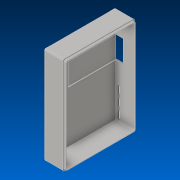
# Autodesk Inventor part: Bottom
Saved by Autodesk Inventor 2016 (Build 200138000, 138)
## iProperties
Created: 2015-08-21
Part Number: Bottom
Material: Generic
Document SubType Name: Modeling
Designer: Moffitt
Density: 1 g/cm^3
Appearance: Default
Author: Moffitt
Autodesk Inventor part; units mm, degrees
ref_plane "YZ Plane" through (0, 0, 0) normal (1, 0, 0) x (0, 1, 0)
ref_plane "XZ Plane" through (0, 0, 0) normal (0, 1, 0) x (-1, 0, 0)
ref_plane "XY Plane" through (0, 0, 0) normal (0, 0, 1) x (1, 0, 0)
sketch "Very Bottom" plane through (0, 0, 0) normal (1, 0, 0) x (0, 1, 0)
  line L0 (98.706, 61.2459) -> (-91.294, 61.2459)
  line L1 (-91.294, 61.2459) -> (-91.294, -78.7541)
  line L2 (-91.294, -78.7541) -> (98.706, -78.7541)
  line L3 (98.706, -78.7541) -> (98.706, 61.2459)
  point P0 (0, 0)
  dimension "d4" = 140
  dimension "d5" = 190
  constraints: 8 end point, 2 parallel, 1 horizontal, 1 perpendicular
  measures "d4" distance of L2.end L0.start
  measures "d5" distance of L1.end L2.end
extrude "Extrusion1" add sketch "Very Bottom" along normal blind 4
sketch "Walls A" plane through (4, 0, 0) normal (1, 0, 0) x (0, 0, -1)
  line L0 (-58.2459, 95.706) -> (75.7541, 95.706)
  line L1 (75.7541, 95.706) -> (75.7541, -88.294)
  line L2 (75.7541, -88.294) -> (-58.2459, -88.294)
  line L3 (-58.2459, -88.294) -> (-58.2459, 95.706)
  line L4 (78.7541, 98.706) -> (-61.2459, 98.706) projected
  line L5 (-61.2459, -91.294) -> (78.7541, -91.294) projected
  line L6 (-61.2459, 98.706) -> (-61.2459, -91.294) projected
  line L7 (78.7541, -91.294) -> (78.7541, 98.706) projected
  point P0 (0, 0)
  dimension "d6" = 3
  dimension "d7" = 3
  dimension "d8" = 3
  dimension "d9" = 3
  constraints: 8 end point, 2 parallel, 1 horizontal, 1 perpendicular
  measures "d6" distance between parallel lines of L4 L0
  measures "d7" distance between parallel lines of L5 L2
  measures "d8" distance between parallel lines of L3 L6
  measures "d9" distance between parallel lines of L7 L1
extrude "Walls" add sketch "Walls A" along normal blind 38
sketch "Back Panel" plane through (0, -91.294, -78.7541) normal (0, 0, -1) x (-1, 0, 0)
  line L0 (0, 0) -> (-42, 0) projected
  line L1 (-4, 3) -> (-4, 187) projected
  line L2 (-4, 103.5669) -> (-19, 103.5669)
  line L3 (-19, 103.5669) -> (-19, 147.5669)
  line L4 (-19, 147.5669) -> (-4, 147.5669)
  line L5 (-4, 147.5669) -> (-4, 103.5669)
  line L6 (-4, 147.5669) -> (0, 147.5669)
  line L7 (0, 147.5669) -> (0, 103.5669)
  line L8 (0, 103.5669) -> (-4, 103.5669)
  line L9 (-4, 103.5669) -> (-4, 147.5669)
  point P0 (0, 91.294)
  dimension "d33" = 44
  dimension "d34" = 15
  dimension "d52" = 4
  constraints: 16 end point, 4 parallel, 2 horizontal, 2 perpendicular, 1 point on line
  measures "d33" distance of L2.end L3.end
  measures "d34" distance of L3.end L4.end
  measures "d52" distance of L4.end L6.end
fillet "Fillet1" radius 3 12 edges at (21, 98.706, -78.7541) (0, 3.706, -78.7541) (21, -91.294, -78.7541) (0, -91.294, -8.7541) (21, -91.294, 61.2459) (0, 3.706, 61.2459) (21, 98.706, 61.2459) (23, 95.706, 58.2459) (23, 95.706, -75.7541) (23, -88.294, -75.7541) (23, -88.294, 58.2459) (0, 98.706, -8.7541)
sketch "Sketch9" plane through (3, 98.706, -75.7541) normal (0, 1, 0) x (1, 0, 0)
  line L0 (-3, 0) -> (-3, -134) projected
  line L1 (-3, -132.5) -> (-1.5, -132.5)
  line L2 (-1.5, -132.5) -> (-1.5, -130.5)
  line L3 (-1.5, -130.5) -> (-3, -130.5)
  line L4 (-3, -130.5) -> (-3, -132.5)
  line L5 (-3, -128.5) -> (-1.5, -128.5)
  line L6 (-1.5, -128.5) -> (-1.5, -126.5)
  line L7 (-1.5, -126.5) -> (-3, -126.5)
  line L8 (-3, -126.5) -> (-3, -128.5)
  line L9 (-3, -1.5) -> (-1.5, -1.5)
  line L10 (-1.5, -1.5) -> (-1.5, -3.5)
  line L11 (-1.5, -3.5) -> (-3, -3.5)
  line L12 (-3, -3.5) -> (-3, -1.5)
  line L13 (-3, -5.5) -> (-1.5, -5.5)
  line L14 (-1.5, -5.5) -> (-1.5, -7.5)
  line L15 (-1.5, -7.5) -> (-3, -7.5)
  line L16 (-3, -7.5) -> (-3, -5.5)
  point P0 (-3, -75.7541)
  dimension "d66" = 1.5
  dimension "d67" = 1.5
  dimension "d68" = 2
  dimension "d69" = 2
  dimension "d70" = 2
  dimension "d71" = 2
  dimension "d72" = 2
  dimension "d73" = 1.5
  dimension "d74" = 2
  dimension "d75" = 1.5
  dimension "d76" = 1.5
  constraints: 32 end point, 8 parallel, 5 point on line, 4 horizontal, 4 perpendicular
  measures "d66" distance of L14.end L15.end
  measures "d67" distance of L10.end L11.end
  measures "d68" distance of L9.end L10.end
  measures "d69" distance of L13.end L14.end
  measures "d70" distance between parallel lines of L11 L13
  measures "d71" distance of L1.end L2.end
  measures "d72" distance of L5.end L6.end
  measures "d73" distance from line of L0.end L1
  measures "d74" distance between parallel lines of L5 L3
  measures "d75" distance of L6.end L7.end
  measures "d76" distance from line of L0.start L9
extrude "Extrusion8" cut sketch "Sketch9" against normal blind 200
extrude "Extrusion9" cut sketch "Back Panel" against normal blind 5 contours L2 L3 L4 L1
fillet "Fillet5" radius 1 1 edges at (11.5, 12.273, -75.7541)
sketch "Sketch11" plane through (42, 95.706, -78.7541) normal (0, 0, -1) x (-1, 0, 0)
  line L0 (34, -181.567) -> (30, -181.567)
  line L1 (30, -181.567) -> (30, -167.567)
  line L2 (30, -167.567) -> (34, -167.567)
  line L3 (34, -167.567) -> (34, -181.567)
  line L4 (30, -160.567) -> (34, -160.567)
  line L5 (34, -160.567) -> (34, -146.567)
  line L6 (34, -146.567) -> (30, -146.567)
  line L7 (30, -146.567) -> (30, -160.567)
  line L8 (30, -139.567) -> (34, -139.567)
  line L9 (34, -139.567) -> (34, -125.567)
  line L10 (34, -125.567) -> (30, -125.567)
  line L11 (30, -125.567) -> (30, -139.567)
  point P0 (42, -95.706)
  dimension "d91" = 14
  dimension "d92" = 4
  dimension "d93" = 7
  dimension "d94" = 14
  dimension "d95" = 4
  dimension "d96" = 7
  dimension "d97" = 14
  dimension "d98" = 4
  constraints: 24 end point, 6 parallel, 3 horizontal, 3 perpendicular
  measures "d91" distance between parallel lines of L2 L0
  measures "d92" distance of L0.start L0.end
  measures "d93" distance between parallel lines of L4 L2
  measures "d94" distance of L6.end L4.start
  measures "d95" distance of L5.end L6.end
  measures "d96" distance between parallel lines of L8 L6
  measures "d97" distance of L10.end L8.start
  measures "d98" distance of L9.end L10.end
extrude "Button Cutous" cut sketch "Sketch11" against normal blind 5
sketch "Button retention slots" plane through (42, -85.294, -75.7541) normal (0, 0, 1) x (1, 0, 0)
  line L0 (-30, -4.067) -> (-34, -4.067)
  line L1 (-34, -4.067) -> (-34, 58.933)
  line L2 (-34, 58.933) -> (-30, 58.933)
  line L3 (-30, 58.933) -> (-30, -4.067)
  line L4 (-34, -0.567) -> (-30, -0.567) projected
  line L5 (-30, 55.433) -> (-34, 55.433) projected
  line L6 (-30, 20.433) -> (-30, 34.433) projected
  point P0 (-42, 85.294)
  dimension "d103" = 3.5
  dimension "d104" = 3.5
  dimension "d105" = 0
  constraints: 8 end point, 2 parallel, 1 horizontal, 1 perpendicular
  measures "d103" distance between parallel lines of L4 L0
  measures "d104" distance between parallel lines of L2 L5
  measures "d105" distance between parallel lines of L6 L3
extrude "Extrusion12" cut sketch "Button retention slots" against normal blind 2
chamfer "Chamfer5" distance 4 angle 10 4 edges at (12, -78.861, -78.7541) (12, -57.861, -78.7541) (12, -36.861, -78.7541) (19, 34.273, -78.7541) measured on face at (12.5, -36.861, -78.7541) measured on face at (12.5, -57.861, -78.7541) measured on face at (19.5, 34.273, -78.7541) measured on face at (12.5, -78.861, -78.7541)
sketch "Sketch15" plane through (42, 0, 0) normal (1, 0, 0) x (0, 0, -1)
  line L0 (78.7541, 98.706) -> (76.7541, 98.706)
  line L1 (76.7541, 98.706) -> (76.7541, -91.294)
  line L2 (76.7541, -91.294) -> (78.7541, -91.294)
  line L3 (78.7541, -91.294) -> (78.7541, 98.706)
  line L4 (78.7541, -89.294) -> (-61.2459, -89.294)
  line L5 (-61.2459, -89.294) -> (-61.2459, -91.294)
  line L6 (-61.2459, -91.294) -> (78.7541, -91.294)
  line L7 (78.7541, -91.294) -> (78.7541, -89.294)
  line L8 (-59.2459, 98.706) -> (-61.2459, 98.706)
  line L9 (-61.2459, 98.706) -> (-61.2459, -91.294)
  line L10 (-61.2459, -91.294) -> (-59.2459, -91.294)
  line L11 (-59.2459, -91.294) -> (-59.2459, 98.706)
  line L12 (78.7541, 98.706) -> (-61.2459, 98.706)
  line L13 (-61.2459, 98.706) -> (-61.2459, 96.706)
  line L14 (-61.2459, 96.706) -> (78.7541, 96.706)
  line L15 (78.7541, 96.706) -> (78.7541, 98.706)
  line L16 (75.7541, 98.706) -> (-58.2459, 98.706) projected
  line L17 (-55.2459, 95.706) -> (72.7541, 95.706) projected
  line L18 (75.7541, 92.706) -> (75.7541, -85.294) projected
  line L19 (72.7541, -88.294) -> (-55.2459, -88.294) projected
  line L20 (-58.2459, -91.294) -> (75.7541, -91.294) projected
  line L21 (-58.2459, -85.294) -> (-58.2459, 92.706) projected
  line L22 (-61.2459, 95.706) -> (-61.2459, -88.294) projected
  point P0 (0, 0)
  dimension "d121" = 0
  dimension "d122" = 1
  dimension "d123" = 1
  dimension "d124" = 0
  dimension "d125" = 0
  dimension "d126" = 1
  dimension "d127" = 0
  dimension "d128" = 0
  dimension "d129" = 1
  dimension "d130" = 0
  dimension "d131" = 0
  dimension "d132" = 0
  dimension "d133" = 0
  constraints: 32 end point, 8 parallel, 4 horizontal, 4 perpendicular, 1 point on line
  measures "d121" distance between parallel lines of L16 L12
  measures "d122" distance between parallel lines of L17 L14
  measures "d123" distance between parallel lines of L18 L1
  measures "d124" distance between parallel lines of L3 L15
  measures "d125" distance between parallel lines of L3 L7
  measures "d126" distance between parallel lines of L19 L4
  measures "d127" distance between parallel lines of L20 L6
  measures "d128" distance between parallel lines of L6 L2
  measures "d129" distance between parallel lines of L21 L11
  measures "d130" distance between parallel lines of L22 L9
  measures "d131" distance between parallel lines of L22 L5
  measures "d132" distance between parallel lines of L20 L10
  measures "d133" distance between parallel lines of L12 L8
extrude "Extrusion14" cut sketch "Sketch15" against normal blind 4 contours L3 L14 L1 L0 | L1 L14 L11 L12 | L3 L4 L1 L14 | L3 L2 L1 L4 | L1 L6 L11 L4 | L14 L9 L8 L11 | L11 L4 L9 L14 | L11 L6 L5 L4
fillet "Fillet6" radius 3 4 edges at (40, 96.706, -76.7541) (40, -89.294, -76.7541) (40, -89.294, 59.2459) (40, 96.706, 59.2459)
sketch "Sketch16" plane through (4, 0, 0) normal (1, 0, 0) x (0, 0, -1)
  line L0 (78.7541, 56.1522) -> (-17.108, 56.1522)
  line L1 (-17.108, 56.1522) -> (-17.108, 12.1522)
  line L2 (-17.108, 12.1522) -> (78.7541, 12.1522)
  line L3 (78.7541, 12.1522) -> (78.7541, 56.1522)
  line L4 (78.7541, 56.273) -> (78.7541, 12.273) projected
  point P0 (0, 0)
  dimension "d137" = 0
  dimension "d138" = 44
  constraints: 8 end point, 2 parallel, 1 horizontal, 1 perpendicular
  measures "d137" distance between parallel lines of L4 L3
  measures "d138" distance between parallel lines of L2 L0
extrude "Extrusion15" cut sketch "Sketch16" against normal blind 2
fillet "Fillet7" radius 2 2 edges at (3, 56.1522, 17.108) (3, 12.1522, 17.108)
body "Solid1"
